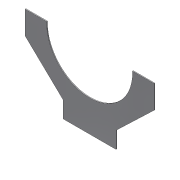
# Autodesk Inventor part: Nema 17 plastic protector
Saved by Autodesk Inventor 2020.2 (Build 242310000, 310)
## iProperties
Created: 2020-01-21
Part Number: Nema 17 plastic protector
Material: Polystyrene
Document SubType Name: Modeling
Designer: james
Density: 1.021 g/cm^3
Appearance: Smooth - White
Mass: 0.0962391 g
Surface Area: 7.85749 cm^2
Volume: 0.0942597 cm^3
Author: james
Autodesk Inventor part; units mm, degrees
ref_plane "YZ Plane" through (0, 0, 0) normal (1, 0, 0) x (0, 1, 0)
ref_plane "XZ Plane" through (0, 0, 0) normal (0, 1, 0) x (-1, 0, 0)
ref_plane "XY Plane" through (0, 0, 0) normal (0, 0, 1) x (1, 0, 0)
sketch "Sketch11" plane through (0, 0, 0) normal (0, 1, 0) x (-1, 0, 0)
  circle A0 centre (0, 0) radius 13
  line L0 (19.5, 0.5) -> (19.5, -6.5)
  line L1 (19.5, -6.5) -> (8, -17.5)
  line L2 (8, -17.5) -> (8, -22.5)
  line L3 (8, -22.5) -> (0, -22.5)
  line L4 (0, -22.5) -> (0, -13)
  line L5 (19.5, 0.5) -> (12.9904, 0.5)
  dimension "d82" = 39
  dimension "d83" = 26
  dimension "d84" = 16
  dimension "d85" = 23
  dimension "d86" = 7
  dimension "d87" = 5
  dimension "d88" = 9.5
  constraints: 12 end point, 3 perpendicular, 2 point on circle, 1 centre point, 1 coincident, 1 parallel, 1 vertical, 1 vertical alignment
  measures "d82" diameter of L0 L4
  measures "d83" diameter of A0
  measures "d84" diameter of L2 L4
  measures "d85" distance between parallel lines of L5 L3
  measures "d86" distance of L0.start L0.end
  measures "d87" distance of L1.end L2.end
  measures "d88" distance of L3.end L4.end
extrude "Extrusion7" add sketch "Sketch11" along normal blind 0.25 contours A0 L5 L0 L1 L2 L3 L4
mirror "Mirror5" about plane through (0, 0, -13) normal (1, 0, 0)
body "Solid6"
